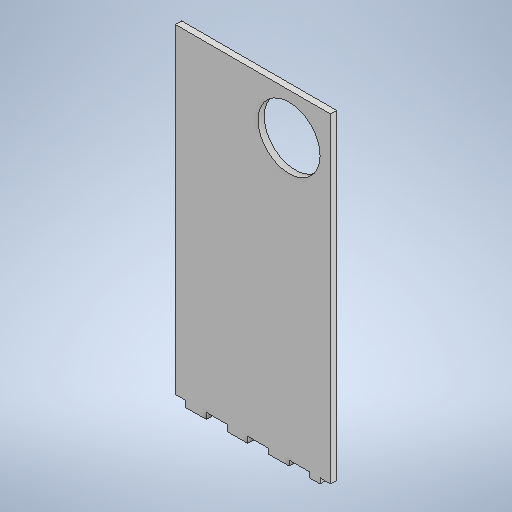
# Autodesk Inventor part: Exit
Saved by Autodesk Inventor 2025.3 (Build 293356000, 356)
## iProperties
Created: 2026-04-16
Part Number: Exit
Material: Generic
Document SubType Name: Modeling
Designer: ziada
Density: 1 g/cm^3
Appearance: Default
Author: ziada
Autodesk Inventor part; units mm, degrees
ref_plane "YZ Plane" through (0, 0, 0) normal (1, 0, 0) x (0, 1, 0)
ref_plane "XZ Plane" through (0, 0, 0) normal (0, 1, 0) x (-1, 0, 0)
ref_plane "XY Plane" through (0, 0, 0) normal (0, 0, 1) x (1, 0, 0)
sketch "Sketch1" plane through (0, 0, 0) normal (0, 0, 1) x (1, 0, 0)
  line L0 (0, 0) -> (0, 6)
  line L1 (0, 6) -> (10, 6)
  line L2 (10, 6) -> (10, 0)
  line L3 (10, 0) -> (30, 0)
  line L4 (30, 0) -> (30, 6)
  line L5 (30, 6) -> (50, 6)
  line L6 (50, 6) -> (50, 0)
  line L7 (50, 0) -> (70, 0)
  line L8 (70, 0) -> (70, 6)
  line L9 (70, 6) -> (90, 6)
  line L10 (90, 6) -> (90, 1)
  line L11 (90, 1) -> (110, 1)
  line L12 (110, 1) -> (110, 6)
  line L13 (110, 6) -> (130, 6)
  line L14 (130, 6) -> (130, 1)
  line L15 (130, 1) -> (140, 1)
  line L16 (140, 1) -> (140, 6)
  line L17 (140, 6) -> (150, 6)
  line L18 (150, 6) -> (150, 316)
  line L19 (150, 316) -> (0, 316)
  line L20 (0, 316) -> (0, 6)
  circle A0 centre (110, 276) radius 30
  dimension "d0" = 6
  dimension "d1" = 10
  dimension "d2" = 20
  dimension "d3" = 20
  dimension "d4" = 20
  dimension "d5" = 20
  dimension "d6" = 20
  dimension "d7" = 20
  dimension "d8" = 10
  dimension "d9" = 10
  dimension "d10" = 310
  dimension "d13" = 60
  dimension "d14" = 40
  dimension "d16" = 40
  constraints: 42 end point, 13 perpendicular, 6 point on line, 3 vertical, 2 parallel, 1 centre point, 1 collinear, 1 horizontal
  measures "d0" distance of L0.start L0.end
  measures "d1" distance of L0.end L1.end
  measures "d2" distance of L2.end L3.end
  measures "d3" distance of L4.end L5.end
  measures "d4" distance of L6.end L7.end
  measures "d5" distance of L8.end L9.end
  measures "d6" distance of L10.end L11.end
  measures "d7" distance of L12.end L13.end
  measures "d8" distance of L14.end L15.end
  measures "d9" distance of L16.end L17.end
  measures "d10" distance of L17.end L18.end
  measures "d13" diameter of A0
  measures "d14" distance from line of L19 A0.centre
  measures "d16" distance from line of L18 A0.centre
extrude "Extrusion1" add sketch "Sketch1" against normal blind 6
body "Solid1"
